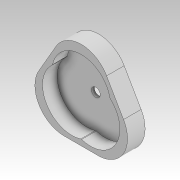
# Autodesk Inventor part: Housing
Saved by Autodesk Inventor 2020 (Build 240168000, 168)
## iProperties
Created: 2021-07-13
Part Number: Housing
Material: Generic
Document SubType Name: Modeling
Designer: DDeGo
Density: 1 g/cm^3
Appearance: Default
Author: DDeGo
Autodesk Inventor part; units mm, degrees
ref_plane "YZ Plane" through (0, 0, 0) normal (1, 0, 0) x (0, 1, 0)
ref_plane "XZ Plane" through (0, 0, 0) normal (0, 1, 0) x (-1, 0, 0)
ref_plane "XY Plane" through (0, 0, 0) normal (0, 0, 1) x (1, 0, 0)
derived "LiquidPistonMasterSketch.ipt"
sketch "Housing" plane through (0, 0, 0) normal (0, 0, 1) x (1, 0, 0)
  circle A0 centre (0, 7.3624) radius 23 construction
  circle A1 centre (0, 7.3624) radius 20 construction
  line L0 (0, 7.3624) -> (0, 0) construction
  circle A2 centre (-6.376, -3.6812) radius 23 construction
  circle A3 centre (-6.376, -3.6812) radius 20 construction
  line L1 (-6.376, -3.6812) -> (0, 0) construction
  circle A4 centre (6.376, -3.6812) radius 23 construction
  circle A5 centre (6.376, -3.6812) radius 20 construction
  line L2 (6.376, -3.6812) -> (0, 0) construction
  line L3 (-19.6048, 11.3188) -> (23.6965, -13.6812) construction
  line L4 (17.3205, 23.3624) -> (28.8927, 3.3188)
  line L5 (11.5722, -26.6812) -> (-11.5722, -26.6812)
  line L6 (-28.8927, 3.3188) -> (-17.3205, 23.3624)
  arc A6 (17.3205, 23.3624) -> (-17.3205, 23.3624) centre (0, 13.3624) ccw
  arc A7 (11.5722, -26.6812) -> (28.8927, 3.3188) centre (11.5722, -6.6812) ccw
  arc A8 (-28.8927, 3.3188) -> (-11.5722, -26.6812) centre (-11.5722, -6.6812) ccw
sketch "RotorCavity" plane through (0, 0, 2) normal (0, 0, 1) x (1, 0, 0)
  arc A0 (19.6048, 11.3188) -> (-19.6048, 11.3188) centre (0, 7.3624) ccw
  arc A1 (0, -22.6376) -> (19.6048, 11.3188) centre (6.376, -3.6812) ccw
  arc A2 (-19.6048, 11.3188) -> (0, -22.6376) centre (-6.376, -3.6812) ccw
  circle A3 centre (0, 7.3624) radius 20 construction
  circle A4 centre (-6.376, -3.6812) radius 20 construction
  circle A5 centre (6.376, -3.6812) radius 20 construction
  circle A6 centre (0, 0) radius 3
  line L0 (0, 0) -> (19.6048, 11.3188) construction
sketch "Sketch4" plane through (0, 0, 2) normal (0, 0, 1) x (1, 0, 0)
  circle A0 centre (0, 0) radius 3
  circle A1 centre (0, 0) radius 5 construction
sketch "Rotor" plane through (0, 0, 2) normal (0, 0, 1) x (1, 0, 0)
  line L0 (-19.6048, 11.3188) -> (23.6965, -13.6812) construction
  arc A0 (9.2104, 17.5845) -> (-10.6234, -16.7687) centre (-2.111, 1.2188) ccw
  arc A1 (-4.9454, -20.0469) -> (14.8884, 14.3063) centre (6.376, -3.6812) ccw
  arc A2 (0, -22.6376) -> (19.6048, 11.3188) centre (6.376, -3.6812) ccw
  circle A3 centre (6.376, -3.6812) radius 20 construction
  line L1 (-19.345, 11.1688) -> (23.6099, -13.6312) construction
  line L2 (-2.111, 1.2188) -> (6.376, -3.6812) construction
  circle A4 centre (2.1325, -1.2312) radius 7.4624 construction
  circle A5 centre (0, 0) radius 5 construction
  line L3 (0, 0) -> (9.8751, 17.1041) construction
  arc A6 (9.2104, 17.5845) -> (14.8884, 14.3063) centre (32.095, 50.6654) ccw
  arc A7 (-4.9454, -20.0469) -> (-10.6234, -16.7687) centre (-27.83, -53.1278) ccw
  line L4 (16.326, 13.5527) -> (7.839, 18.4527) construction
  line L5 (16.6897, 13.1118) -> (9.0734, 17.5091) construction
sketch "RotorBearingPocket" plane through (2.1325, -1.2312, 2) normal (0.8660254, -0.5, 0) x (0.5, 0.8660254, 0)
  line L0 (-69.0165, 3) -> (67.1167, 3) construction
  line L1 (0, 0) -> (0, 3.5)
  line L2 (0, 3.5) -> (8, 3.5) construction
  line L3 (8, 3.5) -> (8, 0)
  line L4 (8, 0) -> (0, 0)
  line L5 (8, 3.5) -> (8.525, 3.5)
  line L6 (8.525, 3.5) -> (8.525, 4)
  line L7 (8.525, 4) -> (9.025, 4)
  line L8 (9.025, 4) -> (9.025, 10)
  line L9 (9.025, 10) -> (0, 10)
  line L10 (0, 10) -> (0, 3.5)
  line L11 (-69.0165, 10) -> (67.1167, 10) construction
  point P0 (0, -2)
ref_plane "BotRotorCavity" through (0, 0, 2) normal (0, 0, 1) x (1, 0, 0)
ref_plane "TopRotorCavity" through (0, 0, 12) normal (0, 0, 1) x (1, 0, 0)
ref_plane "GearsTop" through (0, 0, 5) normal (0, 0, 1) x (1, 0, 0)
ref_plane "RotorCross" through (2.1325, -1.2312, 2) normal (0.8660254, -0.5, 0) x (0.5, 0.8660254, 0)
extrude "Extrusion1" add sketch "Housing" along normal up to surface (12 mm away)
extrude "Extrusion2" cut sketch "RotorCavity" along normal up to surface (10 mm away) contours A1 A2 A0 | A6
extrude "Extrusion3" cut sketch "Sketch4" against normal through all
fillet "Fillet1" radius 1 3 edges at (-19.6048, 11.3188, 7) (19.6048, 11.3188, 7) (0, -22.6376, 7)
body "Solid1"
